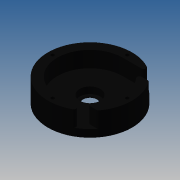
# Autodesk Inventor part: offset shield
Saved by Autodesk Inventor 2013 (Build 170138000, 138)
## iProperties
Created: 2017-03-30
Part Number: offset shield
Material: Generic
Document SubType Name: Modeling
Designer: employee
Density: 1 g/cm^3
Author: employee
Autodesk Inventor part; units mm, degrees
ref_plane "YZ Plane" through (0, 0, 0) normal (1, 0, 0) x (0, 1, 0)
ref_plane "XZ Plane" through (0, 0, 0) normal (0, 1, 0) x (-1, 0, 0)
ref_plane "XY Plane" through (0, 0, 0) normal (0, 0, 1) x (1, 0, 0)
sketch "Sketch1" plane through (0, 0, 0) normal (0, 0, 1) x (1, 0, 0)
  circle A0 centre (0, 0) radius 45
  circle A1 centre (0, 0) radius 35
  dimension "d0" = 90
  dimension "d2" = 70
  constraints: 2 centre point, 2 coincident
  measures "d0" diameter of A0
  measures "d2" diameter of A1
extrude "Extrusion1" add sketch "Sketch1" along normal blind 25
sketch "Sketch2" plane through (0, 0, 0) normal (0, 0, -1) x (-1, 0, 0)
  circle A0 centre (0, 0) radius 35 projected
extrude "Extrusion2" add sketch "Sketch2" against normal blind 8
sketch "Sketch3" plane through (0, 0, 8) normal (0, 0, 1) x (1, 0, 0)
  circle A0 centre (0, 0) radius 35 projected
  circle A1 centre (0, 0) radius 7.5
  dimension "d7" = 15
  constraints: 1 centre point, 1 coincident
  measures "d7" diameter of A1
extrude "Extrusion3" cut sketch "Sketch3" against normal through all contours A1
sketch "Sketch4" plane through (0, 0, 8) normal (0, 0, 1) x (1, 0, 0)
  circle A0 centre (0, 0) radius 7.5 projected
  circle A1 centre (0, 0) radius 35 projected
  circle A2 centre (0, 0) radius 11
  dimension "d11" = 22
  constraints: 1 centre point, 1 coincident
  measures "d11" diameter of A2
extrude "Extrusion4" cut sketch "Sketch4" against normal blind 7 contours A2
sketch "Sketch5" plane through (0, 0, 25) normal (0, 0, 1) x (1, 0, 0)
  circle A0 centre (0, 0) radius 35 construction
  circle A1 centre (0, 0) radius 45 construction
  circle A2 centre (0, 0) radius 32.5 construction
  line L0 (0, 35) -> (35.6195, 35)
  line L1 (35.6195, 35) -> (35.6195, 27.5)
  line L2 (35.6195, 27.5) -> (0, 27.5)
  line L3 (0, 27.5) -> (0, 35)
  line L4 (0, -35) -> (35.6195, -35)
  line L5 (35.6195, -35) -> (35.6195, -27.5)
  line L6 (35.6195, -27.5) -> (0, -27.5)
  line L7 (0, -27.5) -> (0, -35)
  dimension "d15" = 65
  dimension "d17" = 7.5
  constraints: 16 end point, 4 parallel, 4 point on circle, 2 horizontal, 2 perpendicular, 2 tangent, 1 centre point, 1 coincident, 1 collinear
  measures "d15" diameter of A2
  measures "d17" distance of L2.end L0.start
extrude "Extrusion5" cut sketch "Sketch5" against normal up to surface (17 mm away)
fillet "Fillet1" radius 2.5 6 edges at (28.2843, -35, 16.5) (35.6195, -27.5, 16.5) (21.6506, -27.5, 16.5) (21.6506, 27.5, 16.5) (35.6195, 27.5, 16.5) (28.2843, 35, 16.5)
sketch "Sketch6" plane through (0, 0, 0) normal (0, 0, -1) x (-1, 0, 0)
  circle A0 centre (0, 0) radius 7.5 projected
  circle A1 centre (0, 0) radius 45 projected
  circle A2 centre (0, 40) radius 1.75
  dimension "d21" = 40
  dimension "d22" = 3.5
  constraints: 1 centre point, 1 vertical alignment
  measures "d21" distance of A1.centre A2.centre
  measures "d22" diameter of A2
extrude "Extrusion6" cut sketch "Sketch6" against normal through all contours A2
sketch "Sketch7" plane through (0, 0, 0) normal (0, 0, -1) x (-1, 0, 0)
  circle A0 centre (0, 40) radius 1.75 projected
  circle A1 centre (0, 40) radius 3
  dimension "d25" = 6
  constraints: 1 centre point, 1 coincident
  measures "d25" diameter of A1
extrude "Extrusion7" cut sketch "Sketch7" against normal blind 3
pattern_circular "Circular Pattern1" count 4 over 360 about axis through (0, 0, 8) along (0, 0, -1) of "Extrusion7", "Extrusion6"
sketch "Sketch8" plane through (0, 0, 8) normal (0, 0, 1) x (1, 0, 0)
  arc A0 (0, 35) -> (0, -35) centre (0, 0) ccw projected
  circle A1 centre (20, 0) radius 1.75
  dimension "d32" = 20
  dimension "d34" = 3.5
  constraints: 1 centre point, 1 horizontal alignment
  measures "d32" distance of A1.centre A0.centre
  measures "d34" diameter of A1
extrude "Extrusion8" cut sketch "Sketch8" against normal through all
sketch "Sketch9" plane through (0, 0, 8) normal (0, 0, 1) x (1, 0, 0)
  circle A0 centre (20, 0) radius 1.75 projected
  line L0 (20, 3.1754) -> (22.75, 1.5877)
  line L1 (22.75, 1.5877) -> (22.75, -1.5877)
  line L2 (22.75, -1.5877) -> (20, -3.1754)
  line L3 (20, -3.1754) -> (17.25, -1.5877)
  line L4 (17.25, -1.5877) -> (17.25, 1.5877)
  line L5 (17.25, 1.5877) -> (20, 3.1754)
  dimension "d37" = 5.5
  constraints: 12 end point, 1 coincident, 1 vertical, 13 other
  measures "d37" distance between parallel lines of L4 L1
extrude "Extrusion9" cut sketch "Sketch9" against normal blind 4
sketch "Sketch10" plane through (0, 0, 0) normal (0, 0, -1) x (-1, 0, 0)
  circle A0 centre (-40, 0) radius 3 projected
  circle A1 centre (-40, 0) radius 1.75 projected
extrude "Extrusion10" add sketch "Sketch10" against normal up to next
fillet "Fillet2" radius 3.5 1 edges at (-7.5, 0, 1)
body "Solid1"
